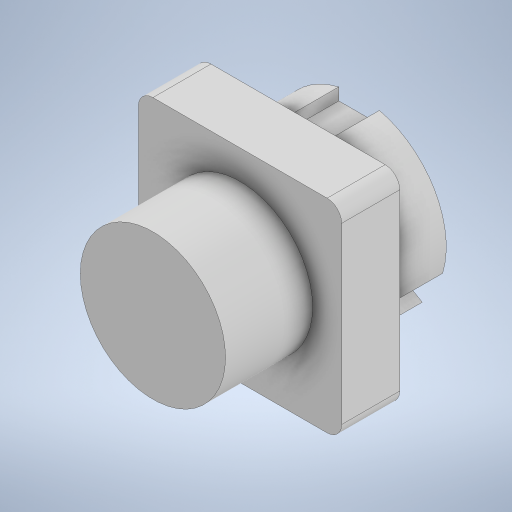
# Autodesk Inventor part: Adapter
Saved by Autodesk Inventor 2023 (Build 270158000, 158)
## iProperties
Created: 2022-09-20
Part Number: Adapter
Material: Generic
Document SubType Name: Modeling
Designer: benni
Density: 1 g/cm^3
Appearance: Default
Author: benni
Autodesk Inventor part; units mm, degrees
ref_plane "YZ Plane" through (0, 0, 0) normal (1, 0, 0) x (0, 1, 0)
ref_plane "XZ Plane" through (0, 0, 0) normal (0, 1, 0) x (-1, 0, 0)
ref_plane "XY Plane" through (0, 0, 0) normal (0, 0, 1) x (1, 0, 0)
sketch "Sketch1" plane through (0, 0, 0) normal (0, 0, 1) x (1, 0, 0)
  circle A0 centre (0, 0) radius 25 construction
  line L0 (0, 0) -> (0, 25) construction
  line L1 (0, 0) -> (21.6506, -12.5) construction
  line L2 (0, 0) -> (-21.6506, -12.5) construction
  line L3 (0, 25) -> (7, 25)
  line L4 (0, 25) -> (-7, 25)
  line L5 (0, 25) -> (7, 25) construction
  line L6 (21.6506, -12.5) -> (25.1506, -6.4378)
  line L7 (21.6506, -12.5) -> (28.6506, -12.5) construction
  line L8 (21.6506, -12.5) -> (18.1506, -18.5622)
  line L9 (21.6506, -12.5) -> (28.6506, -12.5) construction
  line L10 (-21.6506, -12.5) -> (-25.1506, -6.4378)
  line L11 (-21.6506, -12.5) -> (-14.6506, -12.5) construction
  line L12 (-21.6506, -12.5) -> (-18.1506, -18.5622)
  line L13 (-21.6506, -12.5) -> (-14.6506, -12.5) construction
  line L14 (7, 25) -> (7, 29.1719)
  line L15 (-7, 25) -> (-7, 29.1719)
  line L16 (25.1506, -6.4378) -> (28.7636, -8.5238)
  line L17 (18.1506, -18.5622) -> (21.7636, -20.6481)
  line L18 (-18.1506, -18.5622) -> (-21.7636, -20.6481)
  line L19 (-25.1506, -6.4378) -> (-28.7636, -8.5238)
  arc A1 (28.7636, -8.5238) -> (7, 29.1719) centre (0, 0) ccw
  arc A2 (-7, 29.1719) -> (-28.7636, -8.5238) centre (0, 0) ccw
  arc A3 (-21.7636, -20.6481) -> (21.7636, -20.6481) centre (0, 0) ccw
  dimension "d0" = 50
  dimension "d1" = 120
  dimension "d2" = 120
  dimension "d3" = 7
  dimension "d4" = 7
  dimension "d5" = 180
  dimension "d6" = 7
  dimension "d7" = 60
  dimension "d8" = 7
  dimension "d9" = 120
  dimension "d10" = 7
  dimension "d11" = 120
  dimension "d12" = 7
  dimension "d13" = 60
  dimension "d15" = 30
  dimension "d16" = 30
  dimension "d17" = 30
  constraints: 40 end point, 9 point on circle, 6 horizontal, 5 equal length, 4 centre point, 4 tangent, 3 parallel, 2 coincident, 2 vertical, 1 collinear
  measures "d0" diameter of A0
  measures "d1" angle of L1 L0
  measures "d2" angle of L2 L1
  measures "d3" distance of L0.end L3.end
  measures "d4" distance of L0.end L4.end
  measures "d5" angle of L4 L5
  measures "d6" distance of L1.end L6.end
  measures "d7" angle of L7 L6
  measures "d8" distance of L1.end L8.end
  measures "d9" angle of L8 L9
  measures "d10" distance of L2.end L10.end
  measures "d11" angle of L11 L10
  measures "d12" distance of L2.end L12.end
  measures "d13" angle of L12 L13
  measures "d15" radius of A1
  measures "d16" radius of A2
  measures "d17" radius of A3
extrude "Extrusion1" add sketch "Sketch1" along normal blind 21
sketch "Sketch2" plane through (0, 0, 21) normal (0, 0, 1) x (1, 0, 0)
  line L0 (-35, -35) -> (35, -35)
  line L1 (35, -35) -> (35, 35)
  line L2 (35, 35) -> (-35, 35)
  line L3 (-35, 35) -> (-35, -35)
  line L4 (-35, -35) -> (35, 35) construction
  line L5 (35, -35) -> (-35, 35) construction
  point P0 (0, 0)
  dimension "d20" = 70
  dimension "d21" = 70
  constraints: 12 end point, 2 midpoint, 2 parallel, 1 horizontal, 1 perpendicular
  measures "d20" distance of L2.end L1.end
  measures "d21" distance of L1.end L0.end
extrude "Extrusion2" add sketch "Sketch2" along normal blind 20
fillet "Fillet1" radius 5 4 edges at (35, 35, 31) (35, -35, 31) (-35, 35, 31) (-35, -35, 31)
sketch "Sketch3" plane through (0, 0, 41) normal (0, 0, 1) x (1, 0, 0)
  circle A0 centre (0, 0) radius 25
  dimension "d25" = 50
  constraints: 1 centre point, 1 coincident
  measures "d25" diameter of A0
extrude "Extrusion3" add sketch "Sketch3" along normal blind 30
equation "\"d16\" = d15"
equation "\"d17\" = d15"
body "Solid1"
